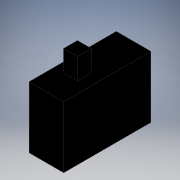
# Autodesk Inventor part: switch
Saved by Autodesk Inventor 2017 (Build 210142000, 142)
## iProperties
Created: 2017-08-03
Part Number: switch
Material: Generic
Document SubType Name: Modeling
Designer: Mitch
Density: 1 g/cm^3
Appearance: Anodized - Black
Author: Mitch
Autodesk Inventor part; units mm, degrees
ref_plane "YZ Plane" through (0, 0, 0) normal (1, 0, 0) x (0, 1, 0)
ref_plane "XZ Plane" through (0, 0, 0) normal (0, 1, 0) x (-1, 0, 0)
ref_plane "XY Plane" through (0, 0, 0) normal (0, 0, 1) x (1, 0, 0)
sketch "Sketch1" plane through (0, 0, 0) normal (0, 1, 0) x (-1, 0, 0)
  line L0 (0, 0) -> (3.5814, 0)
  line L1 (3.5814, 0) -> (3.5814, -9.017)
  line L2 (3.5814, -9.017) -> (0, -9.017)
  line L3 (0, -9.017) -> (0, 0)
  dimension "d0" = 3.5814
  dimension "d1" = 9.017
  constraints: 8 end point, 2 parallel, 1 horizontal, 1 perpendicular
  measures "d0" distance of L1.end L2.end
  measures "d1" distance of L0.end L1.end
extrude "Extrusion1" add sketch "Sketch1" along normal blind 6.35
sketch "Sketch2" plane through (0, 6.35, 0) normal (0, 1, 0) x (1, 0, 0)
  line L0 (-2.6162, 2.5908) -> (-1.1684, 2.5908)
  line L1 (-1.1684, 2.5908) -> (-1.1684, 4.0386)
  line L2 (-1.1684, 4.0386) -> (-2.6162, 4.0386)
  line L3 (-2.6162, 4.0386) -> (-2.6162, 2.5908)
  line L4 (-3.5814, 0) -> (0, 0) projected
  line L5 (0, 0) -> (0, 9.017) projected
  dimension "d4" = 1.4478
  dimension "d5" = 1.4478
  dimension "d6" = 2.5908
  dimension "d7" = 1.1684
  constraints: 8 end point, 2 parallel, 1 horizontal, 1 perpendicular
  measures "d4" distance of L2.end L1.end
  measures "d5" distance of L1.end L0.end
  measures "d6" distance between parallel lines of L4 L0
  measures "d7" distance between parallel lines of L1 L5
extrude "Extrusion2" add sketch "Sketch2" along normal blind 2.159
body "Solid1"
